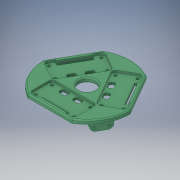
# Autodesk Inventor part: Stewart-Plate-inside
Saved by Autodesk Inventor 2018.2 (Build 222227000, 227)
## iProperties
Created: 2018-02-18
Part Number: Stewart-Plate-inside
Material: Generisch
Document SubType Name: Modeling
Designer: JochenAlt
Density: 1 g/cm^3
Appearance: Vorgabe
Author: JochenAlt
Autodesk Inventor part; units mm, degrees
ref_plane "YZ Plane" through (0, 0, 0) normal (1, 0, 0) x (0, 1, 0)
ref_plane "XZ Plane" through (0, 0, 0) normal (0, 1, 0) x (-1, 0, 0)
ref_plane "XY Plane" through (0, 0, 0) normal (0, 0, 1) x (1, 0, 0)
sketch "Skizze1" plane through (0, 0, 0) normal (0, 0, 1) x (1, 0, 0)
  line L0 (-54.6, 0) -> (54.6, 0) construction
  circle A0 centre (0, 0) radius 39
  line L1 (-8, 36) -> (8, 36)
  line L2 (8, 36) -> (8, 33)
  line L3 (8, 33) -> (-8, 33)
  line L4 (-8, 33) -> (-8, 36)
  line L5 (1.5, 33) -> (-1.5, 33)
  line L6 (-1.5, 33) -> (-1.5, 23)
  line L7 (-1.5, 23) -> (1.5, 23)
  line L8 (1.5, 23) -> (1.5, 33)
  circle A1 centre (0, 0) radius 7.5
  dimension "d9" = 78
  dimension "d10" = 3
  dimension "d11" = 33
  dimension "d14" = 16
  dimension "d23" = 10
  dimension "d62" = 15
  constraints: 16 end point, 4 parallel, 3 perpendicular, 2 centre point, 2 horizontal, 1 coincident, 1 midpoint, 1 point on line
  measures "d9" diameter of A0
  measures "d10" distance between parallel lines of L3 L1
  measures "d11" distance from line of L3 A0.centre
  measures "d14" distance between parallel lines of L2 L4
  measures "d23" distance between parallel lines of L3 L7
  measures "d62" diameter of A1
extrude "Extrusion3" add sketch "Skizze1" against normal blind 7 contours L1 L2 L3 L4 | L3 L8 L7 L6
fillet "Rundung1" radius 4 2 edges at (-8, 34.5, -7) (8, 34.5, -7)
sketch "Skizze2" plane through (-8, 36, 0) normal (0, 1, 0) x (1, 0, 0)
  circle A0 centre (3, 4) radius 1.1
  circle A1 centre (13, 4) radius 1.1
  line L0 (8, 0) -> (8, 7) construction
  line L1 (43, 0) -> (-27, 0) construction
  line L2 (-1.6221, 4) -> (19.0112, 4) construction
  line L3 (4, 7) -> (12, 7) construction
  line L4 (0, 0) -> (0, 3) projected
  dimension "d16" = 2.2
  dimension "d20" = 3
  dimension "d21" = 3
  constraints: 4 end point, 2 centre point, 1 equal radius, 1 horizontal, 1 midpoint, 1 point on line, 1 symmetric about line, 1 vertical
  measures "d16" diameter of A0
  measures "d20" distance between parallel lines of L3 L2
  measures "d21" distance from line of L4 A0.centre
extrude "Extrusion4" cut sketch "Skizze2" against normal up to next
chamfer "Fase1" distance 10 distance2 7 1 edges at (0, 23, -7) measured on face at (0.5, 29.6667, -7)
pattern_circular "Runde Anordnung1" count 3 over 360 about axis through (0, 0, -10) along (0, 0, 1) of "Extrusion3", "Extrusion4", "Fase1", "Rundung1"
sketch "Skizze3" plane through (0, 0, 0) normal (0, 0, 1) x (1, 0, 0)
  line L0 (-11.9, -11.4042) -> (-0.25, -11.4042) construction
  line L1 (-0.25, -11.4042) -> (-0.25, -31.4042) construction
  line L2 (-0.25, -31.4042) -> (-11.9, -31.4042) construction
  line L3 (-11.9, -31.4042) -> (-11.9, -11.4042) construction
  line L4 (0.25, -11.4042) -> (11.9, -11.4042) construction
  line L5 (11.9, -11.4042) -> (11.9, -31.4042) construction
  line L6 (11.9, -31.4042) -> (0.25, -31.4042) construction
  line L7 (0.25, -31.4042) -> (0.25, -11.4042) construction
  line L8 (0, 54.6) -> (0, -54.6) construction
  circle A0 centre (0, 0) radius 16.477 construction
  line L9 (0, 0) -> (14.2695, 8.2385) construction
  line L10 (-11.9, -30.3042) -> (11.9, -30.3042) construction
  line L11 (-11.9, -28.3042) -> (11.9, -28.3042) construction
  line L12 (-12.2, -11.1042) -> (12.2, -11.1042)
  line L13 (12.2, -11.1042) -> (12.2, -31.7042)
  line L14 (12.2, -31.7042) -> (-12.2, -31.7042)
  line L15 (-12.2, -31.7042) -> (-12.2, -11.1042)
  line L16 (-12.2, -30.6042) -> (12.2, -30.6042)
  line L17 (-12.2, -28.0042) -> (12.2, -28.0042)
  line L18 (-9.075, -13.4042) -> (-9.075, -15.4042) construction
  line L19 (-3.075, -13.4042) -> (-3.075, -15.4042) construction
  line L20 (3.075, -13.4042) -> (3.075, -15.4042) construction
  line L21 (9.075, -13.4042) -> (9.075, -15.4042) construction
  line L22 (6.075, -12.4042) -> (6.075, -31.4042) construction
  line L23 (-8.075, -12.4042) -> (-4.075, -12.4042) construction
  line L24 (-8.075, -16.4042) -> (-4.075, -16.4042) construction
  line L25 (4.075, -12.4042) -> (8.075, -12.4042) construction
  line L26 (4.075, -16.4042) -> (8.075, -16.4042) construction
  arc A1 (-8.075, -12.4042) -> (-9.075, -13.4042) centre (-8.075, -13.4042) ccw construction
  arc A2 (-3.075, -13.4042) -> (-4.075, -12.4042) centre (-4.075, -13.4042) ccw construction
  arc A3 (-4.075, -16.4042) -> (-3.075, -15.4042) centre (-4.075, -15.4042) ccw construction
  arc A4 (-9.075, -15.4042) -> (-8.075, -16.4042) centre (-8.075, -15.4042) ccw construction
  arc A5 (3.075, -15.4042) -> (4.075, -16.4042) centre (4.075, -15.4042) ccw construction
  arc A6 (4.075, -12.4042) -> (3.075, -13.4042) centre (4.075, -13.4042) ccw construction
  arc A7 (9.075, -13.4042) -> (8.075, -12.4042) centre (8.075, -13.4042) ccw construction
  arc A8 (8.075, -16.4042) -> (9.075, -15.4042) centre (8.075, -15.4042) ccw construction
  line L27 (-4.075, -16.7042) -> (-8.075, -16.7042)
  arc A9 (-9.375, -15.4042) -> (-8.075, -16.7042) centre (-8.075, -15.4042) ccw
  line L28 (-9.375, -15.4042) -> (-9.375, -13.4076)
  arc A10 (-8.075, -12.1042) -> (-9.375, -13.4076) centre (-8.075, -13.4042) ccw
  line L29 (-8.075, -12.1042) -> (-4.075, -12.1042)
  arc A11 (-2.775, -13.4076) -> (-4.075, -12.1042) centre (-4.075, -13.4042) ccw
  line L30 (-2.775, -13.4076) -> (-2.775, -15.4042)
  arc A12 (-4.075, -16.7042) -> (-2.775, -15.4042) centre (-4.075, -15.4042) ccw
  line L31 (8.075, -12.1042) -> (4.075, -12.1042)
  arc A13 (4.075, -12.1042) -> (2.775, -13.4076) centre (4.075, -13.4042) ccw
  line L32 (2.775, -13.4076) -> (2.775, -15.4076)
  arc A14 (2.775, -15.4076) -> (4.075, -16.7042) centre (4.075, -15.4042) ccw
  line L33 (4.075, -16.7042) -> (8.075, -16.7042)
  arc A15 (8.075, -16.7042) -> (9.375, -15.4076) centre (8.075, -15.4042) ccw
  line L34 (9.375, -15.4076) -> (9.375, -13.4076)
  arc A16 (9.375, -13.4076) -> (8.075, -12.1042) centre (8.075, -13.4042) ccw
  line L35 (-6.075, -11.4042) -> (-6.075, -31.4042) construction
  line L36 (-12.2, -31.7042) -> (-12.2, -32.7042) construction
  circle A17 centre (0, 0) radius 7.5 projected
  line L37 (12.2, -11.1042) -> (17.2, -11.1042)
  line L38 (20.2, -14.1042) -> (20.2, -28.7042)
  line L39 (17.2, -31.7042) -> (12.2, -31.7042)
  line L40 (12.2, -31.7042) -> (12.2, -11.1042)
  line L41 (-12.2, -11.1042) -> (-17.2, -11.1042)
  line L42 (-20.2, -14.1042) -> (-20.2, -28.7042)
  line L43 (-17.2, -31.7042) -> (-12.2, -31.7042)
  line L44 (-12.2, -31.7042) -> (-12.2, -11.1042)
  arc A18 (-17.2, -11.1042) -> (-20.2, -14.1042) centre (-17.2, -14.1042) ccw
  arc A19 (-20.2, -28.7042) -> (-17.2, -31.7042) centre (-17.2, -28.7042) ccw
  arc A20 (20.2, -14.1042) -> (17.2, -11.1042) centre (17.2, -14.1042) ccw
  arc A21 (17.2, -31.7042) -> (20.2, -28.7042) centre (17.2, -28.7042) ccw
  circle A22 centre (17.2, -14.1042) radius 1.3
  circle A23 centre (17.2, -28.7042) radius 1.3
  circle A24 centre (-17.2, -14.1042) radius 1.3
  circle A25 centre (-17.2, -28.7042) radius 1.3
  line L45 (14.2, -11.1042) -> (14.2, -31.7042)
  line L46 (-14.2, -11.1042) -> (-14.2, -31.7042)
  line L47 (15.8264, -4.6036) -> (10.0014, 5.4856) construction
  line L48 (9.7514, 5.9186) -> (3.9264, 16.0078) construction
  line L49 (15.7166, -5.0134) -> (3.5166, 16.1176)
  arc A26 (13.1459, 4.0391) -> (12.7799, 2.6731) centre (13.6459, 3.1731) ccw construction
  arc A27 (12.9989, 4.3006) -> (12.5201, 2.5231) centre (13.6459, 3.1731) ccw
  arc A28 (8.4451, 9.5812) -> (10.2239, 9.107) centre (9.5709, 10.2312) ccw
  arc A29 (8.7049, 9.7312) -> (10.0709, 9.3651) centre (9.5709, 10.2312) ccw construction
  line L50 (6.4451, 13.0453) -> (8.4451, 9.5812)
  line L51 (27.3219, 15.4856) -> (33.1469, 5.3964) construction
  line L52 (21.2469, 26.0078) -> (27.0719, 15.9186) construction
  line L53 (32.1942, 4.8464) -> (20.2942, 25.4578) construction
  line L54 (30.4622, 3.8464) -> (18.5622, 24.4578) construction
  line L55 (21.3567, 26.4176) -> (33.5567, 5.2866)
  line L56 (32.6041, 4.7366) -> (20.4041, 25.8676)
  line L57 (30.3524, 3.4366) -> (18.1524, 24.5676)
  line L58 (33.5567, 5.2866) -> (34.4227, 5.7866) construction
  line L59 (3.9264, 16.0078) -> (21.2469, 26.0078) construction
  line L60 (3.5166, 16.1176) -> (21.3567, 26.4176)
  line L61 (7.0709, 14.5613) -> (8.803, 15.5613) construction
  arc A30 (10.169, 15.1953) -> (8.803, 15.5613) centre (9.303, 14.6953) ccw construction
  arc A31 (7.0709, 14.5613) -> (6.7049, 13.1953) centre (7.5709, 13.6953) ccw construction
  line L62 (8.6559, 15.8228) -> (6.9239, 14.8228)
  arc A32 (10.4288, 15.3453) -> (8.6559, 15.8228) centre (9.303, 14.6953) ccw
  arc A33 (6.9239, 14.8228) -> (6.4451, 13.0453) centre (7.5709, 13.6953) ccw
  line L63 (3.5166, 16.1176) -> (1.0166, 20.4478)
  circle A34 centre (3.6146, 21.9478) radius 1.3
  arc A35 (2.1146, 24.5458) -> (1.0166, 20.4478) centre (3.6146, 21.9478) ccw
  line L64 (7.7049, 11.4632) -> (24.1594, 20.9632) construction
  line L65 (21.3567, 26.4176) -> (3.5166, 16.1176)
  line L66 (2.5166, 17.8497) -> (20.3567, 28.1497)
  line L67 (2.1146, 24.5458) -> (14.7586, 31.8458)
  line L68 (12.4288, 11.8812) -> (10.4288, 15.3453)
  line L69 (12.169, 11.7312) -> (10.169, 15.1953) construction
  line L70 (8.7049, 9.7312) -> (6.7049, 13.1953) construction
  line L71 (18.8567, 30.7478) -> (21.3567, 26.4176)
  circle A36 centre (16.2586, 29.2478) radius 1.3
  arc A37 (18.8567, 30.7478) -> (14.7586, 31.8458) centre (16.2586, 29.2478) ccw
  line L72 (14.7799, -0.791) -> (12.7799, 2.6731) construction
  arc A38 (14.7799, -0.791) -> (16.1459, -1.1571) centre (15.6459, -0.291) ccw construction
  line L73 (14.5201, -0.941) -> (12.5201, 2.5231)
  arc A39 (14.5201, -0.941) -> (16.2989, -1.4152) centre (15.6459, -0.291) ccw
  line L74 (10.0014, 5.4856) -> (27.3219, 15.4856) construction
  line L75 (27.0719, 15.9186) -> (9.7514, 5.9186) construction
  line L76 (12.9139, 0.441) -> (30.2344, 10.441) construction
  line L77 (16.5038, 4.8231) -> (18.5038, 1.359)
  arc A40 (18.028, -0.4169) -> (18.5038, 1.359) centre (17.378, 0.709) ccw
  arc A41 (17.878, -0.1571) -> (18.244, 1.209) centre (17.378, 0.709) ccw construction
  line L78 (18.028, -0.4169) -> (16.2989, -1.4152)
  line L79 (16.1459, -1.1571) -> (17.878, -0.1571) construction
  arc A42 (16.244, 4.6731) -> (14.878, 5.0391) centre (15.378, 4.1731) ccw construction
  arc A43 (16.5038, 4.8231) -> (14.728, 5.2989) centre (15.378, 4.1731) ccw
  line L80 (13.1459, 4.0391) -> (14.878, 5.0391) construction
  line L81 (12.9989, 4.3006) -> (14.728, 5.2989)
  arc A44 (11.9559, 10.107) -> (12.4288, 11.8812) centre (11.303, 11.2312) ccw
  arc A45 (11.803, 10.3651) -> (12.169, 11.7312) centre (11.303, 11.2312) ccw construction
  line L82 (10.2239, 9.107) -> (11.9559, 10.107)
  line L83 (10.0709, 9.3651) -> (11.803, 10.3651) construction
  line L84 (18.244, 1.209) -> (16.244, 4.6731) construction
  line L85 (33.1469, 5.3964) -> (15.8264, -4.6036) construction
  line L86 (33.5567, 5.2866) -> (15.7166, -5.0134)
  line L87 (15.7166, -5.0134) -> (18.2166, -9.3435)
  line L88 (33.5567, 5.2866) -> (15.7166, -5.0134)
  line L89 (16.7166, -6.7454) -> (34.5567, 3.5546)
  line L90 (36.0567, 0.9565) -> (33.5567, 5.2866)
  circle A46 centre (33.4586, -0.5435) radius 1.3
  arc A47 (34.9586, -3.1416) -> (36.0567, 0.9565) centre (33.4586, -0.5435) ccw
  line L91 (22.3146, -10.4416) -> (34.9586, -3.1416)
  circle A48 centre (20.8146, -7.8435) radius 1.3
  arc A49 (18.2166, -9.3435) -> (22.3146, -10.4416) centre (20.8146, -7.8435) ccw
  line L92 (-3.9264, 16.0078) -> (-9.7514, 5.9186) construction
  line L93 (-10.0014, 5.4856) -> (-15.8264, -4.6036) construction
  line L94 (-3.5166, 16.1176) -> (-15.7166, -5.0134)
  arc A50 (-10.0709, 9.3651) -> (-8.7049, 9.7312) centre (-9.5709, 10.2312) ccw construction
  arc A51 (-10.2239, 9.107) -> (-8.4451, 9.5812) centre (-9.5709, 10.2312) ccw
  arc A52 (-12.5201, 2.5231) -> (-12.9989, 4.3006) centre (-13.6459, 3.1731) ccw
  arc A53 (-12.7799, 2.6731) -> (-13.1459, 4.0391) centre (-13.6459, 3.1731) ccw construction
  line L95 (-14.5201, -0.941) -> (-12.5201, 2.5231)
  line L96 (-27.0719, 15.9186) -> (-21.2469, 26.0078) construction
  line L97 (-33.1469, 5.3964) -> (-27.3219, 15.4856) construction
  line L98 (-20.2942, 25.4578) -> (-32.1942, 4.8464) construction
  line L99 (-18.5622, 24.4578) -> (-30.4622, 3.8464) construction
  line L100 (-33.5567, 5.2866) -> (-21.3567, 26.4176)
  line L101 (-20.4041, 25.8676) -> (-32.6041, 4.7366)
  line L102 (-18.1524, 24.5676) -> (-30.3524, 3.4366)
  line L103 (-21.3567, 26.4176) -> (-22.2227, 26.9176) construction
  line L104 (-15.8264, -4.6036) -> (-33.1469, 5.3964) construction
  line L105 (-15.7166, -5.0134) -> (-33.5567, 5.2866)
  line L106 (-16.1459, -1.1571) -> (-17.878, -0.1571) construction
  arc A54 (-18.244, 1.209) -> (-17.878, -0.1571) centre (-17.378, 0.709) ccw construction
  arc A55 (-16.1459, -1.1571) -> (-14.7799, -0.791) centre (-15.6459, -0.291) ccw construction
  line L107 (-18.0309, -0.4152) -> (-16.2989, -1.4152)
  arc A56 (-18.5038, 1.359) -> (-18.0309, -0.4152) centre (-17.378, 0.709) ccw
  arc A57 (-16.2989, -1.4152) -> (-14.5201, -0.941) centre (-15.6459, -0.291) ccw
  line L108 (-15.7166, -5.0134) -> (-18.2166, -9.3435)
  circle A58 centre (-20.8146, -7.8435) radius 1.3
  arc A59 (-22.3146, -10.4416) -> (-18.2166, -9.3435) centre (-20.8146, -7.8435) ccw
  line L109 (-13.7799, 0.941) -> (-30.2344, 10.441) construction
  line L110 (-33.5567, 5.2866) -> (-15.7166, -5.0134)
  line L111 (-16.7166, -6.7454) -> (-34.5567, 3.5546)
  line L112 (-22.3146, -10.4416) -> (-34.9586, -3.1416)
  line L113 (-16.5038, 4.8231) -> (-18.5038, 1.359)
  line L114 (-16.244, 4.6731) -> (-18.244, 1.209) construction
  line L115 (-12.7799, 2.6731) -> (-14.7799, -0.791) construction
  line L116 (-36.0567, 0.9565) -> (-33.5567, 5.2866)
  circle A60 centre (-33.4586, -0.5435) radius 1.3
  arc A61 (-36.0567, 0.9565) -> (-34.9586, -3.1416) centre (-33.4586, -0.5435) ccw
  line L117 (-6.7049, 13.1953) -> (-8.7049, 9.7312) construction
  arc A62 (-6.7049, 13.1953) -> (-7.0709, 14.5613) centre (-7.5709, 13.6953) ccw construction
  line L118 (-6.4451, 13.0453) -> (-8.4451, 9.5812)
  arc A63 (-6.4451, 13.0453) -> (-6.9239, 14.8228) centre (-7.5709, 13.6953) ccw
  line L119 (-9.7514, 5.9186) -> (-27.0719, 15.9186) construction
  line L120 (-27.3219, 15.4856) -> (-10.0014, 5.4856) construction
  line L121 (-6.8389, 10.9632) -> (-24.1594, 20.9632) construction
  line L122 (-12.4288, 11.8812) -> (-10.4288, 15.3453)
  arc A64 (-8.653, 15.8211) -> (-10.4288, 15.3453) centre (-9.303, 14.6953) ccw
  arc A65 (-8.803, 15.5613) -> (-10.169, 15.1953) centre (-9.303, 14.6953) ccw construction
  line L123 (-8.653, 15.8211) -> (-6.9239, 14.8228)
  line L124 (-7.0709, 14.5613) -> (-8.803, 15.5613) construction
  arc A66 (-12.169, 11.7312) -> (-11.803, 10.3651) centre (-11.303, 11.2312) ccw construction
  arc A67 (-12.4288, 11.8812) -> (-11.953, 10.1053) centre (-11.303, 11.2312) ccw
  line L125 (-10.0709, 9.3651) -> (-11.803, 10.3651) construction
  line L126 (-10.2239, 9.107) -> (-11.953, 10.1053)
  arc A68 (-14.7309, 5.3006) -> (-16.5038, 4.8231) centre (-15.378, 4.1731) ccw
  arc A69 (-14.878, 5.0391) -> (-16.244, 4.6731) centre (-15.378, 4.1731) ccw construction
  line L127 (-12.9989, 4.3006) -> (-14.7309, 5.3006)
  line L128 (-13.1459, 4.0391) -> (-14.878, 5.0391) construction
  line L129 (-10.169, 15.1953) -> (-12.169, 11.7312) construction
  line L130 (-21.2469, 26.0078) -> (-3.9264, 16.0078) construction
  line L131 (-21.3567, 26.4176) -> (-3.5166, 16.1176)
  line L132 (-3.5166, 16.1176) -> (-1.0166, 20.4478)
  line L133 (-21.3567, 26.4176) -> (-3.5166, 16.1176)
  line L134 (-2.5166, 17.8497) -> (-20.3567, 28.1497)
  line L135 (-18.8567, 30.7478) -> (-21.3567, 26.4176)
  circle A70 centre (-16.2586, 29.2478) radius 1.3
  arc A71 (-14.7586, 31.8458) -> (-18.8567, 30.7478) centre (-16.2586, 29.2478) ccw
  line L136 (-2.1146, 24.5458) -> (-14.7586, 31.8458)
  circle A72 centre (-3.6146, 21.9478) radius 1.3
  arc A73 (-1.0166, 20.4478) -> (-2.1146, 24.5458) centre (-3.6146, 21.9478) ccw
  line L137 (18.8662, -10.1247) -> (17.1231, -11.1052) construction
  circle A74 centre (0, 0) radius 39 construction
  line L138 (19.0746, -33.7042) -> (-19.0746, -33.7042)
  line L139 (38.726, 0.333) -> (19.6514, 33.3712)
  line L140 (-19.3777, 33.8453) -> (-38.726, 0.333)
  arc A75 (-38.9937, -0.703) -> (-20.1057, -33.418) centre (0, 0) ccw
  arc A76 (20.1057, -33.418) -> (38.9937, -0.703) centre (0, 0) ccw
  arc A77 (18.888, 34.121) -> (-19.3777, 33.8453) centre (0, 0) ccw
  arc A78 (19.0746, -33.7042) -> (20.1057, -33.418) centre (19.0746, -31.7042) ccw
  arc A79 (-20.1057, -33.418) -> (-19.0746, -33.7042) centre (-19.0746, -31.7042) ccw
  arc A80 (-38.726, 0.333) -> (-38.9937, -0.703) centre (-36.994, -0.667) ccw
  arc A81 (38.9937, -0.703) -> (38.726, 0.333) centre (36.994, -0.667) ccw
  arc A82 (19.6514, 33.3712) -> (18.888, 34.121) centre (17.9194, 32.3712) ccw
  point P0 (19.622, -33.7042)
  point P1 (-19.622, -33.7042)
  point P2 (38.9997, -0.1411)
  point P3 (19.3777, 33.8453)
  point P4 (-38.9997, -0.1411)
  dimension "d36" = 11.65
  dimension "d37" = 0.5
  dimension "d38" = 20
  dimension "d40" = 60
  dimension "d41" = 16.9
  dimension "d42" = 2
  dimension "d43" = 0.3
  dimension "d44" = 0.3
  dimension "d45" = 0.3
  dimension "d46" = 0.3
  dimension "d47" = 0.3
  dimension "d48" = 0.3
  dimension "d51" = 6
  dimension "d52" = 1
  dimension "d53" = 5
  dimension "d54" = 1
  dimension "d55" = 0.3
  dimension "d56" = 0.3
  dimension "d61" = 1
  dimension "d67" = 3
  dimension "d68" = 2.6
  dimension "d70" = 2
  dimension "d71" = 8
  dimension "d74" = 360
  dimension "d77" = 2
  dimension "d79" = 2
  dimension "d80" = 2
  dimension "d81" = 2
  dimension "d82" = 2
  dimension "d83" = 39
  constraints: 280 end point, 143 point on circle, 80 centre point, 41 point on line, 34 tangent, 23 perpendicular, 19 equal radius, 14 coincident, 13 parallel, 7 collinear, 7 horizontal, 6 midpoint, 1 vertical, 493 other
  measures "d36" distance between parallel lines of L5 L7
  measures "d37" distance between parallel lines of L7 L1
  measures "d38" distance between parallel lines of L4 L6
  measures "d40" angle of L9 L8
  measures "d41" distance between parallel lines of L11 L4
  measures "d42" distance between parallel lines of L10 L11
  measures "d43" distance between parallel lines of L4 L12
  measures "d44" distance between parallel lines of L5 L13
  measures "d45" distance between parallel lines of L14 L6
  measures "d46" distance between parallel lines of L3 L15
  measures "d47" distance between parallel lines of L11 L17
  measures "d48" distance between parallel lines of L16 L10
  measures "d51" distance between parallel lines of L21 L20
  measures "d52" distance between parallel lines of L4 L25
  measures "d53" distance between parallel lines of L26 L4
  measures "d54" radius of A1
  measures "d55" distance between parallel lines of L27 L24
  measures "d56" distance between parallel lines of L33 L26
  measures "d61" distance of L14.end L36.end
  measures "d67" radius of A18
  measures "d68" diameter of A22
  measures "d70" distance between parallel lines of L13 L45
  measures "d71" distance between parallel lines of L38 L13
  measures "d77" distance of L137.start L137.end
  measures "d79" distance between parallel lines of L14 L138
  measures "d80" distance between parallel lines of L55 L139
  measures "d81" distance between parallel lines of L140 L100
  measures "d82" radius of A78
  measures "d83" radius of A76
extrude "Extrusion6" add sketch "Skizze3" along normal blind 4 contours L16 L13 L14 L15 | L56 L60 L55 L86 | L101 L105 L100 L131 | L138 A79 A75 A80 L140 A77 A82 L139 A81 A76 A78
extrude "Extrusion7" add sketch "Skizze3" along normal blind 2 contours L12 L13 L17 L15 | L15 L43 L46 L41 | L37 L45 L39 L13 | L46 L43 A19 L42 A18 L41 | L37 A20 L38 A21 L39 L45 | L16 L13 L14 L15 | L49 L60 L57 L86 | L86 L90 L89 L87 | L63 L66 L71 L60 | L89 L90 A47 L91 A49 L87 | L63 A35 L67 A37 L71 L66 | L56 L60 L55 L86 | L94 L105 L102 L131 | L131 L135 L134 L132 | L108 L111 L116 L105 | L134 L135 A71 L136 A73 L132 | L108 A59 L112 A61 L116 L111 | L101 L105 L100 L131
fillet "Rundung4" radius 1 24 edges at (-7.5, 0, 4) (-7.5, 0, 0) (19.3208, 33.7981, 4) (29.1887, 16.8521, 4) (38.9304, -0.1668, 4) (33.775, -19.5, 4) (19.6096, -33.6313, 4) (0, -33.7042, 4) (-19.6096, -33.6313, 4) (-33.775, -19.5, 4) (-38.9304, -0.1668, 4) (-29.0519, 17.0892, 4) (-0.281, 38.999, 4) (19.3208, 33.7981, 0) (29.1887, 16.8521, 0) (38.9304, -0.1668, 0) (33.775, -19.5, 0) (19.6096, -33.6313, 0) (0, -33.7042, 0) (-19.6096, -33.6313, 0) (-33.775, -19.5, 0) (-38.9304, -0.1668, 0) (-29.0519, 17.0892, 0) (-0.281, 38.999, 0)
equation "\"d21\" = d20"
equation "\"d44\" = d43"
equation "\"d45\" = d43"
equation "\"d46\" = d43"
equation "\"d47\" = d43"
equation "\"d48\" = d43"
equation "\"d55\" = d43"
equation "\"d56\" = d43"
